Autodesk Inventor part; units mm, degrees
(part 4 of 5)
  line L745 (-387.1432, 38.3282) -> (-386.5943, 38.3282)
  spline S682 degree 2 poles (-383.8413, 38.4244) (-383.8923, 38.447) (-384.0677, 38.4838) (-384.1243, 38.4838) knots 0 0 0 1 2 2 2
  spline S683 degree 2 poles (-384.1243, 38.4838) (-384.5741, 38.4838) (-384.5741, 37.9661) knots 0 0 0 1 1 1
  line L746 (-384.5741, 37.9661) -> (-384.5741, 37.0211)
  line L747 (-384.5741, 37.0211) -> (-385.4795, 37.0211)
  line L748 (-385.4795, 37.0211) -> (-385.4795, 39.1996)
  line L749 (-385.4795, 39.1996) -> (-384.5741, 39.1996)
  line L750 (-384.5741, 39.1996) -> (-384.5741, 38.8177)
  line L751 (-384.5741, 38.8177) -> (-384.5657, 38.8177)
  spline S684 degree 2 poles (-384.5657, 38.8177) (-384.4836, 39.0242) (-384.1752, 39.2392) (-383.9715, 39.2392) knots 0 0 0 1 2 2 2
  spline S685 degree 2 poles (-383.9715, 39.2392) (-383.8979, 39.2392) (-383.8413, 39.2138) knots 0 0 0 1 1 1
  line L752 (-383.8413, 39.2138) -> (-383.8413, 38.4244)
  spline S686 degree 2 poles (-381.9429, 38.4244) (-381.9938, 38.447) (-382.1692, 38.4838) (-382.2258, 38.4838) knots 0 0 0 1 2 2 2
  spline S687 degree 2 poles (-382.2258, 38.4838) (-382.6757, 38.4838) (-382.6757, 37.9661) knots 0 0 0 1 1 1
  line L753 (-382.6757, 37.9661) -> (-382.6757, 37.0211)
  line L754 (-382.6757, 37.0211) -> (-383.5811, 37.0211)
  line L755 (-383.5811, 37.0211) -> (-383.5811, 39.1996)
  line L756 (-383.5811, 39.1996) -> (-382.6757, 39.1996)
  line L757 (-382.6757, 39.1996) -> (-382.6757, 38.8177)
  line L758 (-382.6757, 38.8177) -> (-382.6672, 38.8177)
  spline S688 degree 2 poles (-382.6672, 38.8177) (-382.5851, 39.0242) (-382.2767, 39.2392) (-382.073, 39.2392) knots 0 0 0 1 2 2 2
  spline S689 degree 2 poles (-382.073, 39.2392) (-381.9995, 39.2392) (-381.9429, 39.2138) knots 0 0 0 1 1 1
  line L759 (-381.9429, 39.2138) -> (-381.9429, 38.4244)
  spline S690 degree 2 poles (-379.2607, 38.15) (-379.2607, 37.5982) (-379.9256, 36.9673) (-380.5226, 36.9673) knots 0 0 0 1 2 2 2
  spline S691 degree 2 poles (-380.5226, 36.9673) (-381.1167, 36.9673) (-381.7788, 37.5813) (-381.7788, 38.1245) knots 0 0 0 1 2 2 2
  spline S692 degree 2 poles (-381.7788, 38.1245) (-381.7788, 38.4697) (-381.4676, 38.9818) (-380.8932, 39.2534) (-380.5197, 39.2534) knots 0 0 0 1 2 3 3 3
  spline S693 degree 2 poles (-380.5197, 39.2534) (-380.1321, 39.2534) (-379.5634, 38.9676) (-379.2607, 38.4612) (-379.2607, 38.15) knots 0 0 0 1 2 3 3 3
  spline S694 degree 2 poles (-380.1802, 38.1443) (-380.1802, 38.5885) (-380.5197, 38.5885) knots 0 0 0 1 1 1
  spline S695 degree 2 poles (-380.5197, 38.5885) (-380.8593, 38.5885) (-380.8593, 38.1245) knots 0 0 0 1 1 1
  spline S696 degree 2 poles (-380.8593, 38.1245) (-380.8593, 37.6322) (-380.5141, 37.6322) knots 0 0 0 1 1 1
  spline S697 degree 2 poles (-380.5141, 37.6322) (-380.1802, 37.6322) (-380.1802, 38.1443) knots 0 0 0 1 1 1
  line L760 (-380.6272, 39.5448) -> (-381.3855, 40.2267)
  line L761 (-381.3855, 40.2267) -> (-380.6244, 40.2267)
  line L762 (-380.6244, 40.2267) -> (-379.9878, 39.5448)
  line L763 (-379.9878, 39.5448) -> (-380.6272, 39.5448)
  line L764 (-376.7086, 39.3524) -> (-376.7086, 38.8035)
  line L765 (-376.7086, 38.8035) -> (-375.8033, 38.8035)
  line L766 (-375.8033, 38.8035) -> (-375.8033, 38.0849)
  line L767 (-375.8033, 38.0849) -> (-376.7086, 38.0849)
  line L768 (-376.7086, 38.0849) -> (-376.7086, 37.0211)
  line L769 (-376.7086, 37.0211) -> (-377.6282, 37.0211)
  line L770 (-377.6282, 37.0211) -> (-377.6282, 40.0711)
  line L771 (-377.6282, 40.0711) -> (-375.7156, 40.0711)
  line L772 (-375.7156, 40.0711) -> (-375.7156, 39.3524)
  line L773 (-375.7156, 39.3524) -> (-376.7086, 39.3524)
  spline S698 degree 2 poles (-373.7152, 38.4244) (-373.7662, 38.447) (-373.9416, 38.4838) (-373.9982, 38.4838) knots 0 0 0 1 2 2 2
  spline S699 degree 2 poles (-373.9982, 38.4838) (-374.448, 38.4838) (-374.448, 37.9661) knots 0 0 0 1 1 1
  line L774 (-374.448, 37.9661) -> (-374.448, 37.0211)
  line L775 (-374.448, 37.0211) -> (-375.3534, 37.0211)
  line L776 (-375.3534, 37.0211) -> (-375.3534, 39.1996)
  line L777 (-375.3534, 39.1996) -> (-374.448, 39.1996)
  line L778 (-374.448, 39.1996) -> (-374.448, 38.8177)
  line L779 (-374.448, 38.8177) -> (-374.4395, 38.8177)
  spline S700 degree 2 poles (-374.4395, 38.8177) (-374.3575, 39.0242) (-374.0491, 39.2392) (-373.8454, 39.2392) knots 0 0 0 1 2 2 2
  spline S701 degree 2 poles (-373.8454, 39.2392) (-373.7718, 39.2392) (-373.7152, 39.2138) knots 0 0 0 1 1 1
  line L780 (-373.7152, 39.2138) -> (-373.7152, 38.4244)
  line L781 (-372.2468, 37.0211) -> (-372.2468, 37.3521)
  line L782 (-372.2468, 37.3521) -> (-372.2553, 37.3521)
  spline S702 degree 2 poles (-372.2553, 37.3521) (-372.4732, 36.9673) (-372.9202, 36.9673) knots 0 0 0 1 1 1
  spline S703 degree 2 poles (-372.9202, 36.9673) (-373.2286, 36.9673) (-373.5766, 37.3323) (-373.5766, 37.6407) knots 0 0 0 1 2 2 2
  spline S704 degree 2 poles (-373.5766, 37.6407) (-373.5766, 38.2829) (-372.7872, 38.3848) knots 0 0 0 1 1 1
  line L783 (-372.7872, 38.3848) -> (-372.2468, 38.4555)
  spline S705 degree 2 poles (-372.2468, 38.4555) (-372.2468, 38.563) (-372.4392, 38.6988) (-372.6005, 38.6988) knots 0 0 0 1 2 2 2
  spline S706 degree 2 poles (-372.6005, 38.6988) (-372.9655, 38.6988) (-373.3729, 38.4895) knots 0 0 0 1 1 1
  line L784 (-373.3729, 38.4895) -> (-373.3729, 39.078)
  spline S707 degree 2 poles (-373.3729, 39.078) (-373.1975, 39.1544) (-372.6627, 39.2534) (-372.4732, 39.2534) knots 0 0 0 1 2 2 2
  spline S708 degree 2 poles (-372.4732, 39.2534) (-371.9186, 39.2534) (-371.4178, 38.7781) (-371.4178, 38.2235) knots 0 0 0 1 2 2 2
  line L785 (-371.4178, 38.2235) -> (-371.4178, 37.0211)
  line L786 (-371.4178, 37.0211) -> (-372.2468, 37.0211)
  spline S709 degree 2 poles (-372.7844, 37.7623) (-372.7844, 37.6746) (-372.6712, 37.5586) (-372.5665, 37.5586) knots 0 0 0 1 2 2 2
  spline S710 degree 2 poles (-372.5665, 37.5586) (-372.4251, 37.5586) (-372.2468, 37.7708) (-372.2468, 37.9378) knots 0 0 0 1 2 2 2
  line L787 (-372.2468, 37.9378) -> (-372.2468, 38.0198)
  line L788 (-372.2468, 38.0198) -> (-372.5552, 37.9774)
  spline S711 degree 2 poles (-372.5552, 37.9774) (-372.7844, 37.9378) (-372.7844, 37.7623) knots 0 0 0 1 1 1
  line L789 (-369.5986, 37.0211) -> (-369.5986, 38.2094)
  spline S712 degree 2 poles (-369.5986, 38.2094) (-369.5986, 38.4131) (-369.7202, 38.5885) (-369.8561, 38.5885) knots 0 0 0 1 2 2 2
  spline S713 degree 2 poles (-369.8561, 38.5885) (-369.9721, 38.5885) (-370.105, 38.4046) (-370.105, 38.2631) knots 0 0 0 1 2 2 2
  line L790 (-370.105, 38.2631) -> (-370.105, 37.0211)
  line L791 (-370.105, 37.0211) -> (-371.0104, 37.0211)
  line L792 (-371.0104, 37.0211) -> (-371.0104, 39.1996)
  line L793 (-371.0104, 39.1996) -> (-370.105, 39.1996)
  line L794 (-370.105, 39.1996) -> (-370.105, 38.8601)
  line L795 (-370.105, 38.8601) -> (-370.0965, 38.8601)
  spline S714 degree 2 poles (-370.0965, 38.8601) (-369.989, 39.0469) (-369.6212, 39.2534) (-369.4062, 39.2534) knots 0 0 0 1 2 2 2
  spline S715 degree 2 poles (-369.4062, 39.2534) (-368.6932, 39.2534) (-368.6932, 38.3508) knots 0 0 0 1 1 1
  line L796 (-368.6932, 38.3508) -> (-368.6932, 37.0211)
  line L797 (-368.6932, 37.0211) -> (-369.5986, 37.0211)
  spline S716 degree 2 poles (-366.4892, 37.0833) (-366.5769, 37.0324) (-366.9503, 36.9673) (-367.1937, 36.9673) knots 0 0 0 1 2 2 2
  spline S717 degree 2 poles (-367.1937, 36.9673) (-367.5388, 36.9673) (-368.0821, 37.2474) (-368.3791, 37.7482) (-368.3791, 38.0622) knots 0 0 0 1 2 3 3 3
  spline S718 degree 2 poles (-368.3791, 38.0622) (-368.3791, 38.4357) (-368.0623, 38.9705) (-367.4766, 39.2534) (-367.089, 39.2534) knots 0 0 0 1 2 3 3 3
  spline S719 degree 2 poles (-367.089, 39.2534) (-366.8768, 39.2534) (-366.5373, 39.1968) (-366.4892, 39.1629) knots 0 0 0 1 2 2 2
  line L798 (-366.4892, 39.1629) -> (-366.4892, 38.4555)
  spline S720 degree 2 poles (-366.4892, 38.4555) (-366.5571, 38.5093) (-366.8117, 38.5885) (-366.9192, 38.5885) knots 0 0 0 1 2 2 2
  spline S721 degree 2 poles (-366.9192, 38.5885) (-367.1852, 38.5885) (-367.4596, 38.3367) (-367.4596, 38.1075) knots 0 0 0 1 2 2 2
  spline S722 degree 2 poles (-367.4596, 38.1075) (-367.4596, 37.8812) (-367.1908, 37.6322) (-366.9532, 37.6322) knots 0 0 0 1 2 2 2
  spline S723 degree 2 poles (-366.9532, 37.6322) (-366.7014, 37.6322) (-366.4892, 37.751) knots 0 0 0 1 1 1
  line L799 (-366.4892, 37.751) -> (-366.4892, 37.0833)
  spline S724 degree 2 poles (-365.3461, 37.8529) (-365.3235, 37.7114) (-365.0462, 37.553) (-364.8199, 37.553) knots 0 0 0 1 2 2 2
  spline S725 degree 2 poles (-364.8199, 37.553) (-364.503, 37.553) (-364.2201, 37.6746) knots 0 0 0 1 1 1
  line L800 (-364.2201, 37.6746) -> (-364.2201, 37.1003)
  spline S726 degree 2 poles (-364.2201, 37.1003) (-364.5483, 36.9673) (-365.0208, 36.9673) knots 0 0 0 1 1 1
  spline S727 degree 2 poles (-365.0208, 36.9673) (-365.5894, 36.9673) (-366.2232, 37.5501) (-366.2232, 38.0622) knots 0 0 0 1 2 2 2
  spline S728 degree 2 poles (-366.2232, 38.0622) (-366.2232, 38.4131) (-365.9459, 38.9478) (-365.3999, 39.2534) (-365.0689, 39.2534) knots 0 0 0 1 2 3 3 3
  spline S729 degree 2 poles (-365.0689, 39.2534) (-364.7322, 39.2534) (-364.2512, 38.9903) (-364.0022, 38.5121) (-364.0022, 38.1924) knots 0 0 0 1 2 3 3 3
  line L801 (-364.0022, 38.1924) -> (-364.0022, 37.8529)
  line L802 (-364.0022, 37.8529) -> (-365.3461, 37.8529)
  spline S730 degree 2 poles (-364.8029, 38.3282) (-364.8029, 38.7045) (-365.0717, 38.7045) knots 0 0 0 1 1 1
  spline S731 degree 2 poles (-365.0717, 38.7045) (-365.1849, 38.7045) (-365.3376, 38.498) (-365.3518, 38.3282) knots 0 0 0 1 2 2 2
  line L803 (-365.3518, 38.3282) -> (-364.8029, 38.3282)
  spline S732 degree 2 poles (-361.917, 37.7454) (-361.917, 37.3747) (-362.4829, 36.9673) (-362.9865, 36.9673) knots 0 0 0 1 2 2 2
  spline S733 degree 2 poles (-362.9865, 36.9673) (-363.1336, 36.9673) (-363.5665, 37.0267) (-363.7023, 37.0692) knots 0 0 0 1 2 2 2
  line L804 (-363.7023, 37.0692) -> (-363.7023, 37.7058)
  spline S734 degree 2 poles (-363.7023, 37.7058) (-363.3005, 37.5275) (-363.0289, 37.5275) knots 0 0 0 1 1 1
  spline S735 degree 2 poles (-363.0289, 37.5275) (-362.763, 37.5275) (-362.763, 37.6661) knots 0 0 0 1 1 1
  spline S736 degree 2 poles (-362.763, 37.6661) (-362.763, 37.7227) (-362.8875, 37.7991) (-363.1477, 37.884) knots 0 0 0 1 2 2 2
  spline S737 degree 2 poles (-363.1477, 37.884) (-363.4392, 37.9774) (-363.7023, 38.2801) (-363.7023, 38.5206) knots 0 0 0 1 2 2 2
  spline S738 degree 2 poles (-363.7023, 38.5206) (-363.7023, 38.8601) (-363.1619, 39.2534) (-362.6753, 39.2534) knots 0 0 0 1 2 2 2
  spline S739 degree 2 poles (-362.6753, 39.2534) (-362.3895, 39.2534) (-362.0698, 39.1713) knots 0 0 0 1 1 1
  line L805 (-362.0698, 39.1713) -> (-362.0698, 38.5602)
  spline S740 degree 2 poles (-362.0698, 38.5602) (-362.2056, 38.6168) (-362.5253, 38.6932) (-362.6328, 38.6932) knots 0 0 0 1 2 2 2
  spline S741 degree 2 poles (-362.6328, 38.6932) (-362.7234, 38.6932) (-362.8309, 38.6338) (-362.8309, 38.58) knots 0 0 0 1 2 2 2
  spline S742 degree 2 poles (-362.8309, 38.58) (-362.8309, 38.5178) (-362.7149, 38.4414) (-362.5423, 38.3876) knots 0 0 0 1 2 2 2
  spline S743 degree 2 poles (-362.5423, 38.3876) (-362.2084, 38.2914) (-361.917, 37.9859) (-361.917, 37.7454) knots 0 0 0 1 2 2 2
  spline S744 degree 2 poles (-359.7894, 37.0833) (-359.8771, 37.0324) (-360.2505, 36.9673) (-360.4939, 36.9673) knots 0 0 0 1 2 2 2
  spline S745 degree 2 poles (-360.4939, 36.9673) (-360.839, 36.9673) (-361.3823, 37.2474) (-361.6793, 37.7482) (-361.6793, 38.0622) knots 0 0 0 1 2 3 3 3
  spline S746 degree 2 poles (-361.6793, 38.0622) (-361.6793, 38.4357) (-361.3625, 38.9705) (-360.7768, 39.2534) (-360.3892, 39.2534) knots 0 0 0 1 2 3 3 3
  spline S747 degree 2 poles (-360.3892, 39.2534) (-360.177, 39.2534) (-359.8375, 39.1968) (-359.7894, 39.1629) knots 0 0 0 1 2 2 2
  line L806 (-359.7894, 39.1629) -> (-359.7894, 38.4555)
  spline S748 degree 2 poles (-359.7894, 38.4555) (-359.8573, 38.5093) (-360.1119, 38.5885) (-360.2194, 38.5885) knots 0 0 0 1 2 2 2
  spline S749 degree 2 poles (-360.2194, 38.5885) (-360.4854, 38.5885) (-360.7598, 38.3367) (-360.7598, 38.1075) knots 0 0 0 1 2 2 2
  spline S750 degree 2 poles (-360.7598, 38.1075) (-360.7598, 37.8812) (-360.491, 37.6322) (-360.2534, 37.6322) knots 0 0 0 1 2 2 2
  spline S751 degree 2 poles (-360.2534, 37.6322) (-360.0016, 37.6322) (-359.7894, 37.751) knots 0 0 0 1 1 1
  line L807 (-359.7894, 37.751) -> (-359.7894, 37.0833)
  spline S752 degree 2 poles (-357.0053, 38.15) (-357.0053, 37.5982) (-357.6702, 36.9673) (-358.2672, 36.9673) knots 0 0 0 1 2 2 2
  spline S753 degree 2 poles (-358.2672, 36.9673) (-358.8613, 36.9673) (-359.5234, 37.5813) (-359.5234, 38.1245) knots 0 0 0 1 2 2 2
  spline S754 degree 2 poles (-359.5234, 38.1245) (-359.5234, 38.4697) (-359.2122, 38.9818) (-358.6378, 39.2534) (-358.2644, 39.2534) knots 0 0 0 1 2 3 3 3
  spline S755 degree 2 poles (-358.2644, 39.2534) (-357.8767, 39.2534) (-357.308, 38.9676) (-357.0053, 38.4612) (-357.0053, 38.15) knots 0 0 0 1 2 3 3 3
  spline S756 degree 2 poles (-357.9248, 38.1443) (-357.9248, 38.5885) (-358.2644, 38.5885) knots 0 0 0 1 1 1
  spline S757 degree 2 poles (-358.2644, 38.5885) (-358.6039, 38.5885) (-358.6039, 38.1245) knots 0 0 0 1 1 1
  spline S758 degree 2 poles (-358.6039, 38.1245) (-358.6039, 37.6322) (-358.2587, 37.6322) knots 0 0 0 1 1 1
  spline S759 degree 2 poles (-358.2587, 37.6322) (-357.9248, 37.6322) (-357.9248, 38.1443) knots 0 0 0 1 1 1
  spline S760 degree 2 poles (-268.9959, 67.4041) (-268.9959, 66.9542) (-269.6268, 66.4676) (-270.2097, 66.4676) knots 0 0 0 1 2 2 2
  line L808 (-270.2097, 66.4676) -> (-271.6017, 66.4676)
  line L809 (-271.6017, 66.4676) -> (-271.6017, 69.5176)
  line L810 (-271.6017, 69.5176) -> (-270.3059, 69.5176)
  spline S761 degree 2 poles (-270.3059, 69.5176) (-269.0921, 69.5176) (-269.0921, 68.7791) knots 0 0 0 1 1 1
  spline S762 degree 2 poles (-269.0921, 68.7791) (-269.0921, 68.6207) (-269.2449, 68.3547) (-269.5589, 68.1539) (-269.7457, 68.1171) knots 0 0 0 1 2 3 3 3
  line L811 (-269.7457, 68.1171) -> (-269.7457, 68.1086)
  spline S763 degree 2 poles (-269.7457, 68.1086) (-269.5278, 68.0831) (-269.1826, 67.8766) (-268.9959, 67.5682) (-268.9959, 67.4041) knots 0 0 0 1 2 3 3 3
  spline S764 degree 2 poles (-269.972, 67.4069) (-269.972, 67.5399) (-270.1644, 67.7097) (-270.32, 67.7097) knots 0 0 0 1 2 2 2
  line L812 (-270.32, 67.7097) -> (-270.6822, 67.7097)
  line L813 (-270.6822, 67.7097) -> (-270.6822, 67.0872)
  line L814 (-270.6822, 67.0872) -> (-270.3766, 67.0872)
  spline S765 degree 2 poles (-270.3766, 67.0872) (-270.1899, 67.0872) (-269.972, 67.2598) (-269.972, 67.4069) knots 0 0 0 1 2 2 2
  spline S766 degree 2 poles (-270.0682, 68.6207) (-270.0682, 68.9036) (-270.5124, 68.9036) knots 0 0 0 1 1 1
  line L815 (-270.5124, 68.9036) -> (-270.6822, 68.9036)
  line L816 (-270.6822, 68.9036) -> (-270.6822, 68.3264)
  line L817 (-270.6822, 68.3264) -> (-270.4162, 68.3264)
  spline S767 degree 2 poles (-270.4162, 68.3264) (-270.2634, 68.3264) (-270.0682, 68.4905) (-270.0682, 68.6207) knots 0 0 0 1 2 2 2
  spline S768 degree 2 poles (-266.2515, 67.5965) (-266.2515, 67.0448) (-266.9163, 66.4138) (-267.5133, 66.4138) knots 0 0 0 1 2 2 2
  spline S769 degree 2 poles (-267.5133, 66.4138) (-268.1075, 66.4138) (-268.7695, 67.0278) (-268.7695, 67.571) knots 0 0 0 1 2 2 2
  spline S770 degree 2 poles (-268.7695, 67.571) (-268.7695, 67.9162) (-268.4583, 68.4283) (-267.884, 68.6999) (-267.5105, 68.6999) knots 0 0 0 1 2 3 3 3
  spline S771 degree 2 poles (-267.5105, 68.6999) (-267.1229, 68.6999) (-266.5542, 68.4142) (-266.2515, 67.9077) (-266.2515, 67.5965) knots 0 0 0 1 2 3 3 3
  spline S772 degree 2 poles (-267.171, 67.5908) (-267.171, 68.035) (-267.5105, 68.035) knots 0 0 0 1 1 1
  spline S773 degree 2 poles (-267.5105, 68.035) (-267.85, 68.035) (-267.85, 67.571) knots 0 0 0 1 1 1
  spline S774 degree 2 poles (-267.85, 67.571) (-267.85, 67.0787) (-267.5048, 67.0787) knots 0 0 0 1 1 1
  spline S775 degree 2 poles (-267.5048, 67.0787) (-267.171, 67.0787) (-267.171, 67.5908) knots 0 0 0 1 1 1
  line L818 (-264.7038, 66.4676) -> (-264.7038, 66.7986)
  line L819 (-264.7038, 66.7986) -> (-264.7123, 66.7986)
  spline S776 degree 2 poles (-264.7123, 66.7986) (-264.9302, 66.4138) (-265.3772, 66.4138) knots 0 0 0 1 1 1
  spline S777 degree 2 poles (-265.3772, 66.4138) (-265.6856, 66.4138) (-266.0336, 66.7788) (-266.0336, 67.0872) knots 0 0 0 1 2 2 2
  spline S778 degree 2 poles (-266.0336, 67.0872) (-266.0336, 67.7295) (-265.2442, 67.8313) knots 0 0 0 1 1 1
  line L820 (-265.2442, 67.8313) -> (-264.7038, 67.902)
  spline S779 degree 2 poles (-264.7038, 67.902) (-264.7038, 68.0096) (-264.8962, 68.1454) (-265.0575, 68.1454) knots 0 0 0 1 2 2 2
  spline S780 degree 2 poles (-265.0575, 68.1454) (-265.4225, 68.1454) (-265.8299, 67.936) knots 0 0 0 1 1 1
  line L821 (-265.8299, 67.936) -> (-265.8299, 68.5245)
  spline S781 degree 2 poles (-265.8299, 68.5245) (-265.6545, 68.6009) (-265.1197, 68.6999) (-264.9302, 68.6999) knots 0 0 0 1 2 2 2
  spline S782 degree 2 poles (-264.9302, 68.6999) (-264.3756, 68.6999) (-263.8748, 68.2246) (-263.8748, 67.67) knots 0 0 0 1 2 2 2
  line L822 (-263.8748, 67.67) -> (-263.8748, 66.4676)
  line L823 (-263.8748, 66.4676) -> (-264.7038, 66.4676)
  spline S783 degree 2 poles (-265.2414, 67.2089) (-265.2414, 67.1212) (-265.1282, 67.0052) (-265.0235, 67.0052) knots 0 0 0 1 2 2 2
  spline S784 degree 2 poles (-265.0235, 67.0052) (-264.8821, 67.0052) (-264.7038, 67.2174) (-264.7038, 67.3843) knots 0 0 0 1 2 2 2
  line L824 (-264.7038, 67.3843) -> (-264.7038, 67.4663)
  line L825 (-264.7038, 67.4663) -> (-265.0122, 67.4239)
  spline S785 degree 2 poles (-265.0122, 67.4239) (-265.2414, 67.3843) (-265.2414, 67.2089) knots 0 0 0 1 1 1
  spline S786 degree 2 poles (-261.8292, 67.8709) (-261.8802, 67.8936) (-262.0556, 67.9303) (-262.1122, 67.9303) knots 0 0 0 1 2 2 2
  spline S787 degree 2 poles (-262.1122, 67.9303) (-262.562, 67.9303) (-262.562, 67.4126) knots 0 0 0 1 1 1
  line L826 (-262.562, 67.4126) -> (-262.562, 66.4676)
  line L827 (-262.562, 66.4676) -> (-263.4674, 66.4676)
  line L828 (-263.4674, 66.4676) -> (-263.4674, 68.6462)
  line L829 (-263.4674, 68.6462) -> (-262.562, 68.6462)
  line L830 (-262.562, 68.6462) -> (-262.562, 68.2642)
  line L831 (-262.562, 68.2642) -> (-262.5535, 68.2642)
  spline S788 degree 2 poles (-262.5535, 68.2642) (-262.4715, 68.4707) (-262.1631, 68.6858) (-261.9594, 68.6858) knots 0 0 0 1 2 2 2
  spline S789 degree 2 poles (-261.9594, 68.6858) (-261.8858, 68.6858) (-261.8292, 68.6603) knots 0 0 0 1 1 1
  line L832 (-261.8292, 68.6603) -> (-261.8292, 67.8709)
  line L833 (-260.1147, 66.4676) -> (-260.1147, 66.7222)
  line L834 (-260.1147, 66.7222) -> (-260.1232, 66.7222)
  spline S790 degree 2 poles (-260.1232, 66.7222) (-260.2307, 66.5779) (-260.5815, 66.4138) (-260.7513, 66.4138) knots 0 0 0 1 2 2 2
  spline S791 degree 2 poles (-260.7513, 66.4138) (-261.0285, 66.4138) (-261.4558, 66.6883) (-261.6651, 67.1834) (-261.6651, 67.5173) knots 0 0 0 1 2 3 3 3
  spline S792 degree 2 poles (-261.6651, 67.5173) (-261.6651, 67.8653) (-261.4133, 68.4028) (-260.9578, 68.6999) (-260.6749, 68.6999) knots 0 0 0 1 2 3 3 3
  spline S793 degree 2 poles (-260.6749, 68.6999) (-260.5419, 68.6999) (-260.3156, 68.6235) (-260.1458, 68.4934) (-260.1232, 68.4283) knots 0 0 0 1 2 3 3 3
  line L835 (-260.1232, 68.4283) -> (-260.1147, 68.4283)
  line L836 (-260.1147, 68.4283) -> (-260.1147, 69.693)
  line L837 (-260.1147, 69.693) -> (-259.2093, 69.693)
  line L838 (-259.2093, 69.693) -> (-259.2093, 66.4676)
  line L839 (-259.2093, 66.4676) -> (-260.1147, 66.4676)
  spline S794 degree 2 poles (-260.0949, 67.6219) (-260.0949, 67.8172) (-260.2675, 68.035) (-260.4146, 68.035) knots 0 0 0 1 2 2 2
  spline S795 degree 2 poles (-260.4146, 68.035) (-260.5617, 68.035) (-260.7456, 67.7662) (-260.7456, 67.5399) knots 0 0 0 1 2 2 2
  spline S796 degree 2 poles (-260.7456, 67.5399) (-260.7456, 67.0787) (-260.4259, 67.0787) knots 0 0 0 1 1 1
  spline S797 degree 2 poles (-260.4259, 67.0787) (-260.2759, 67.0787) (-260.0949, 67.3277) (-260.0949, 67.5654) knots 0 0 0 1 2 2 2
  line L840 (-260.0949, 67.5654) -> (-260.0949, 67.6219)
  line L841 (-255.4774, 66.4619) -> (-255.6557, 66.6713)
  spline S798 degree 2 poles (-255.6557, 66.6713) (-255.7971, 66.5609) (-256.3121, 66.4138) (-256.5469, 66.4138) knots 0 0 0 1 2 2 2
  spline S799 degree 2 poles (-256.5469, 66.4138) (-257.0675, 66.4138) (-257.6475, 66.8665) (-257.6475, 67.2739) knots 0 0 0 1 2 2 2
  spline S800 degree 2 poles (-257.6475, 67.2739) (-257.6475, 67.5144) (-257.2995, 67.953) (-256.9402, 68.1312) knots 0 0 0 1 2 2 2
  spline S801 degree 2 poles (-256.9402, 68.1312) (-257.2458, 68.4679) (-257.2458, 68.8018) knots 0 0 0 1 1 1
  spline S802 degree 2 poles (-257.2458, 68.8018) (-257.2458, 69.1441) (-256.711, 69.5685) (-256.2838, 69.5685) knots 0 0 0 1 2 2 2
  spline S803 degree 2 poles (-256.2838, 69.5685) (-255.8764, 69.5685) (-255.3812, 69.1866) (-255.3812, 68.8697) knots 0 0 0 1 2 2 2
  spline S804 degree 2 poles (-255.3812, 68.8697) (-255.3812, 68.6179) (-255.6755, 68.2529) (-255.9924, 68.1058) knots 0 0 0 1 2 2 2
  line L842 (-255.9924, 68.1058) -> (-255.5595, 67.6135)
  spline S805 degree 2 poles (-255.5595, 67.6135) (-255.4633, 67.8058) (-255.4633, 68.1312) knots 0 0 0 1 1 1
  line L843 (-255.4633, 68.1312) -> (-254.7701, 68.1312)
  spline S806 degree 2 poles (-254.7701, 68.1312) (-254.7701, 67.8228) (-254.9455, 67.3305) (-255.1407, 67.1268) knots 0 0 0 1 2 2 2
  line L844 (-255.1407, 67.1268) -> (-254.5296, 66.4619)
  line L845 (-254.5296, 66.4619) -> (-255.4774, 66.4619)
  spline S807 degree 2 poles (-256.6205, 67.7606) (-256.711, 67.7181) (-256.8327, 67.5088) (-256.8327, 67.3786) knots 0 0 0 1 2 2 2
  spline S808 degree 2 poles (-256.8327, 67.3786) (-256.8327, 67.1975) (-256.5922, 66.9769) (-256.4168, 66.9769) knots 0 0 0 1 2 2 2
  spline S809 degree 2 poles (-256.4168, 66.9769) (-256.3093, 66.9769) (-256.1055, 67.0476) (-256.0376, 67.1042) knots 0 0 0 1 2 2 2
  line L846 (-256.0376, 67.1042) -> (-256.6205, 67.7606)
  spline S810 degree 2 poles (-256.0801, 68.8244) (-256.0801, 68.9149) (-256.2131, 69.0451) (-256.3036, 69.0451) knots 0 0 0 1 2 2 2
  spline S811 degree 2 poles (-256.3036, 69.0451) (-256.4111, 69.0451) (-256.5384, 68.9291) (-256.5384, 68.8272) knots 0 0 0 1 2 2 2
  spline S812 degree 2 poles (-256.5384, 68.8272) (-256.5384, 68.7622) (-256.4592, 68.6235) (-256.3177, 68.4622) knots 0 0 0 1 2 2 2
  spline S813 degree 2 poles (-256.3177, 68.4622) (-256.1848, 68.5443) (-256.0801, 68.7141) (-256.0801, 68.8244) knots 0 0 0 1 2 2 2
  spline S814 degree 2 poles (-250.7779, 66.5496) (-251.1571, 66.4138) (-251.6522, 66.4138) knots 0 0 0 1 1 1
  spline S815 degree 2 poles (-251.6522, 66.4138) (-252.1388, 66.4138) (-252.8433, 66.7873) (-253.2168, 67.472) (-253.2168, 67.9218) knots 0 0 0 1 2 3 3 3
  spline S816 degree 2 poles (-253.2168, 67.9218) (-253.2168, 68.4057) (-252.8009, 69.1583) (-252.0398, 69.5685) (-251.5447, 69.5685) knots 0 0 0 1 2 3 3 3
  spline S817 degree 2 poles (-251.5447, 69.5685) (-251.1486, 69.5685) (-250.7779, 69.4723) knots 0 0 0 1 1 1
  line L847 (-250.7779, 69.4723) -> (-250.7779, 68.6235)
  spline S818 degree 2 poles (-250.7779, 68.6235) (-250.9053, 68.6999) (-251.2589, 68.7848) (-251.4372, 68.7848) knots 0 0 0 1 2 2 2
  spline S819 degree 2 poles (-251.4372, 68.7848) (-251.8135, 68.7848) (-252.2435, 68.3547) (-252.2435, 67.9869) knots 0 0 0 1 2 2 2
  spline S820 degree 2 poles (-252.2435, 67.9869) (-252.2435, 67.6219) (-251.8135, 67.1975) (-251.4513, 67.1975) knots 0 0 0 1 2 2 2
  spline S821 degree 2 poles (-251.4513, 67.1975) (-251.1175, 67.1975) (-250.7779, 67.3701) knots 0 0 0 1 1 1
  line L848 (-250.7779, 67.3701) -> (-250.7779, 66.5496)
  line L849 (-249.1766, 66.4676) -> (-249.1766, 66.7986)
  line L850 (-249.1766, 66.7986) -> (-249.185, 66.7986)
  spline S822 degree 2 poles (-249.185, 66.7986) (-249.4029, 66.4138) (-249.8499, 66.4138) knots 0 0 0 1 1 1
  spline S823 degree 2 poles (-249.8499, 66.4138) (-250.1583, 66.4138) (-250.5063, 66.7788) (-250.5063, 67.0872) knots 0 0 0 1 2 2 2
  spline S824 degree 2 poles (-250.5063, 67.0872) (-250.5063, 67.7295) (-249.717, 67.8313) knots 0 0 0 1 1 1
  line L851 (-249.717, 67.8313) -> (-249.1766, 67.902)
  spline S825 degree 2 poles (-249.1766, 67.902) (-249.1766, 68.0096) (-249.3689, 68.1454) (-249.5302, 68.1454) knots 0 0 0 1 2 2 2
  spline S826 degree 2 poles (-249.5302, 68.1454) (-249.8952, 68.1454) (-250.3026, 67.936) knots 0 0 0 1 1 1
  line L852 (-250.3026, 67.936) -> (-250.3026, 68.5245)
  spline S827 degree 2 poles (-250.3026, 68.5245) (-250.1272, 68.6009) (-249.5925, 68.6999) (-249.4029, 68.6999) knots 0 0 0 1 2 2 2
  spline S828 degree 2 poles (-249.4029, 68.6999) (-248.8484, 68.6999) (-248.3476, 68.2246) (-248.3476, 67.67) knots 0 0 0 1 2 2 2
  line L853 (-248.3476, 67.67) -> (-248.3476, 66.4676)
  line L854 (-248.3476, 66.4676) -> (-249.1766, 66.4676)
  spline S829 degree 2 poles (-249.7141, 67.2089) (-249.7141, 67.1212) (-249.6009, 67.0052) (-249.4963, 67.0052) knots 0 0 0 1 2 2 2
  spline S830 degree 2 poles (-249.4963, 67.0052) (-249.3548, 67.0052) (-249.1766, 67.2174) (-249.1766, 67.3843) knots 0 0 0 1 2 2 2
  line L855 (-249.1766, 67.3843) -> (-249.1766, 67.4663)
  line L856 (-249.1766, 67.4663) -> (-249.4849, 67.4239)
  spline S831 degree 2 poles (-249.4849, 67.4239) (-249.7141, 67.3843) (-249.7141, 67.2089) knots 0 0 0 1 1 1
  spline S832 degree 2 poles (-246.169, 67.1919) (-246.169, 66.8212) (-246.7349, 66.4138) (-247.2385, 66.4138) knots 0 0 0 1 2 2 2
  spline S833 degree 2 poles (-247.2385, 66.4138) (-247.3856, 66.4138) (-247.8185, 66.4732) (-247.9543, 66.5157) knots 0 0 0 1 2 2 2
  line L857 (-247.9543, 66.5157) -> (-247.9543, 67.1523)
  spline S834 degree 2 poles (-247.9543, 67.1523) (-247.5525, 66.974) (-247.2809, 66.974) knots 0 0 0 1 1 1
  spline S835 degree 2 poles (-247.2809, 66.974) (-247.015, 66.974) (-247.015, 67.1127) knots 0 0 0 1 1 1
  spline S836 degree 2 poles (-247.015, 67.1127) (-247.015, 67.1693) (-247.1394, 67.2456) (-247.3997, 67.3305) knots 0 0 0 1 2 2 2
  spline S837 degree 2 poles (-247.3997, 67.3305) (-247.6912, 67.4239) (-247.9543, 67.7266) (-247.9543, 67.9671) knots 0 0 0 1 2 2 2
  spline S838 degree 2 poles (-247.9543, 67.9671) (-247.9543, 68.3066) (-247.4139, 68.6999) (-246.9272, 68.6999) knots 0 0 0 1 2 2 2
  spline S839 degree 2 poles (-246.9272, 68.6999) (-246.6415, 68.6999) (-246.3218, 68.6179) knots 0 0 0 1 1 1
  line L858 (-246.3218, 68.6179) -> (-246.3218, 68.0067)
  spline S840 degree 2 poles (-246.3218, 68.0067) (-246.4576, 68.0633) (-246.7773, 68.1397) (-246.8848, 68.1397) knots 0 0 0 1 2 2 2
  spline S841 degree 2 poles (-246.8848, 68.1397) (-246.9753, 68.1397) (-247.0829, 68.0803) (-247.0829, 68.0265) knots 0 0 0 1 2 2 2
  spline S842 degree 2 poles (-247.0829, 68.0265) (-247.0829, 67.9643) (-246.9669, 67.8879) (-246.7943, 67.8341) knots 0 0 0 1 2 2 2
  spline S843 degree 2 poles (-246.7943, 67.8341) (-246.4604, 67.7379) (-246.169, 67.4324) (-246.169, 67.1919) knots 0 0 0 1 2 2 2
  spline S844 degree 2 poles (-245.0542, 67.2994) (-245.0316, 67.1579) (-244.7543, 66.9995) (-244.528, 66.9995) knots 0 0 0 1 2 2 2
  spline S845 degree 2 poles (-244.528, 66.9995) (-244.2111, 66.9995) (-243.9282, 67.1212) knots 0 0 0 1 1 1
  line L859 (-243.9282, 67.1212) -> (-243.9282, 66.5468)
  spline S846 degree 2 poles (-243.9282, 66.5468) (-244.2564, 66.4138) (-244.7289, 66.4138) knots 0 0 0 1 1 1
  spline S847 degree 2 poles (-244.7289, 66.4138) (-245.2976, 66.4138) (-245.9313, 66.9967) (-245.9313, 67.5088) knots 0 0 0 1 2 2 2
  spline S848 degree 2 poles (-245.9313, 67.5088) (-245.9313, 67.8596) (-245.6541, 68.3943) (-245.108, 68.6999) (-244.777, 68.6999) knots 0 0 0 1 2 3 3 3
  spline S849 degree 2 poles (-244.777, 68.6999) (-244.4403, 68.6999) (-243.9593, 68.4368) (-243.7103, 67.9586) (-243.7103, 67.6389) knots 0 0 0 1 2 3 3 3
  line L860 (-243.7103, 67.6389) -> (-243.7103, 67.2994)
  line L861 (-243.7103, 67.2994) -> (-245.0542, 67.2994)
  spline S850 degree 2 poles (-244.511, 67.7747) (-244.511, 68.151) (-244.7798, 68.151) knots 0 0 0 1 1 1
  spline S851 degree 2 poles (-244.7798, 68.151) (-244.893, 68.151) (-245.0458, 67.9445) (-245.0599, 67.7747) knots 0 0 0 1 2 2 2
  line L862 (-245.0599, 67.7747) -> (-244.511, 67.7747)
  spline S852 degree 2 poles (-239.2259, 68.0322) (-239.2259, 67.5682) (-239.6163, 66.8552) (-240.3378, 66.4676) (-240.8103, 66.4676) knots 0 0 0 1 2 3 3 3
  line L863 (-240.8103, 66.4676) -> (-242.1033, 66.4676)
  line L864 (-242.1033, 66.4676) -> (-242.1033, 69.5176)
  line L865 (-242.1033, 69.5176) -> (-240.8386, 69.5176)
  spline S853 degree 2 poles (-240.8386, 69.5176) (-239.2259, 69.5176) (-239.2259, 68.0322) knots 0 0 0 1 1 1
  spline S854 degree 2 poles (-240.202, 68.0237) (-240.202, 68.2444) (-240.383, 68.6037) (-240.7197, 68.7989) (-240.9461, 68.7989) knots 0 0 0 1 2 3 3 3
  line L866 (-240.9461, 68.7989) -> (-241.1837, 68.7989)
  line L867 (-241.1837, 68.7989) -> (-241.1837, 67.1862)
  line L868 (-241.1837, 67.1862) -> (-240.9263, 67.1862)
  spline S855 degree 2 poles (-240.9263, 67.1862) (-240.5952, 67.1862) (-240.202, 67.6389) (-240.202, 68.0237) knots 0 0 0 1 2 2 2
  spline S856 degree 2 poles (-238.097, 67.2994) (-238.0743, 67.1579) (-237.7971, 66.9995) (-237.5707, 66.9995) knots 0 0 0 1 2 2 2
  spline S857 degree 2 poles (-237.5707, 66.9995) (-237.2538, 66.9995) (-236.9709, 67.1212) knots 0 0 0 1 1 1
  line L869 (-236.9709, 67.1212) -> (-236.9709, 66.5468)
  spline S858 degree 2 poles (-236.9709, 66.5468) (-237.2991, 66.4138) (-237.7716, 66.4138) knots 0 0 0 1 1 1
  spline S859 degree 2 poles (-237.7716, 66.4138) (-238.3403, 66.4138) (-238.974, 66.9967) (-238.974, 67.5088) knots 0 0 0 1 2 2 2
  spline S860 degree 2 poles (-238.974, 67.5088) (-238.974, 67.8596) (-238.6968, 68.3943) (-238.1507, 68.6999) (-237.8197, 68.6999) knots 0 0 0 1 2 3 3 3
  spline S861 degree 2 poles (-237.8197, 68.6999) (-237.483, 68.6999) (-237.002, 68.4368) (-236.753, 67.9586) (-236.753, 67.6389) knots 0 0 0 1 2 3 3 3
  line L870 (-236.753, 67.6389) -> (-236.753, 67.2994)
  line L871 (-236.753, 67.2994) -> (-238.097, 67.2994)
  spline S862 degree 2 poles (-237.5537, 67.7747) (-237.5537, 68.151) (-237.8225, 68.151) knots 0 0 0 1 1 1
  spline S863 degree 2 poles (-237.8225, 68.151) (-237.9357, 68.151) (-238.0885, 67.9445) (-238.1026, 67.7747) knots 0 0 0 1 2 2 2
  line L872 (-238.1026, 67.7747) -> (-237.5537, 67.7747)
  line L873 (-234.8546, 66.4676) -> (-235.9297, 66.4676)
  line L874 (-235.9297, 66.4676) -> (-236.6568, 68.6462)
  line L875 (-236.6568, 68.6462) -> (-235.7118, 68.6462)
  line L876 (-235.7118, 68.6462) -> (-235.4459, 67.4578)
  spline S864 degree 2 poles (-235.4459, 67.4578) (-235.3836, 67.1693) (-235.3752, 67.025) knots 0 0 0 1 1 1
  line L877 (-235.3752, 67.025) -> (-235.3638, 67.025)
  spline S865 degree 2 poles (-235.3638, 67.025) (-235.3582, 67.0674) (-235.344, 67.1579) (-235.0356, 68.6462) knots 0 0 0 1 2 2 2
  line L878 (-235.0356, 68.6462) -> (-234.0963, 68.6462)
  line L879 (-234.0963, 68.6462) -> (-234.8546, 66.4676)
  spline S866 degree 2 poles (-233.0976, 67.2994) (-233.0749, 67.1579) (-232.7977, 66.9995) (-232.5713, 66.9995) knots 0 0 0 1 2 2 2
  spline S867 degree 2 poles (-232.5713, 66.9995) (-232.2544, 66.9995) (-231.9715, 67.1212) knots 0 0 0 1 1 1
  line L880 (-231.9715, 67.1212) -> (-231.9715, 66.5468)
  spline S868 degree 2 poles (-231.9715, 66.5468) (-232.2997, 66.4138) (-232.7722, 66.4138) knots 0 0 0 1 1 1
  spline S869 degree 2 poles (-232.7722, 66.4138) (-233.3409, 66.4138) (-233.9746, 66.9967) (-233.9746, 67.5088) knots 0 0 0 1 2 2 2
  spline S870 degree 2 poles (-233.9746, 67.5088) (-233.9746, 67.8596) (-233.6974, 68.3943) (-233.1513, 68.6999) (-232.8203, 68.6999) knots 0 0 0 1 2 3 3 3
  spline S871 degree 2 poles (-232.8203, 68.6999) (-232.4836, 68.6999) (-232.0026, 68.4368) (-231.7536, 67.9586) (-231.7536, 67.6389) knots 0 0 0 1 2 3 3 3
  line L881 (-231.7536, 67.6389) -> (-231.7536, 67.2994)
  line L882 (-231.7536, 67.2994) -> (-233.0976, 67.2994)
  spline S872 degree 2 poles (-232.5543, 67.7747) (-232.5543, 68.151) (-232.8231, 68.151) knots 0 0 0 1 1 1
  spline S873 degree 2 poles (-232.8231, 68.151) (-232.9363, 68.151) (-233.0891, 67.9445) (-233.1032, 67.7747) knots 0 0 0 1 2 2 2
  line L883 (-233.1032, 67.7747) -> (-232.5543, 67.7747)
  line L884 (-231.4396, 66.4676) -> (-231.4396, 69.693)
  line L885 (-231.4396, 69.693) -> (-230.5342, 69.693)
  line L886 (-230.5342, 69.693) -> (-230.5342, 66.4676)
  line L887 (-230.5342, 66.4676) -> (-231.4396, 66.4676)
  spline S874 degree 2 poles (-227.6766, 67.5965) (-227.6766, 67.0448) (-228.3415, 66.4138) (-228.9385, 66.4138) knots 0 0 0 1 2 2 2
  spline S875 degree 2 poles (-228.9385, 66.4138) (-229.5326, 66.4138) (-230.1947, 67.0278) (-230.1947, 67.571) knots 0 0 0 1 2 2 2
  spline S876 degree 2 poles (-230.1947, 67.571) (-230.1947, 67.9162) (-229.8835, 68.4283) (-229.3091, 68.6999) (-228.9356, 68.6999) knots 0 0 0 1 2 3 3 3
  spline S877 degree 2 poles (-228.9356, 68.6999) (-228.548, 68.6999) (-227.9793, 68.4142) (-227.6766, 67.9077) (-227.6766, 67.5965) knots 0 0 0 1 2 3 3 3
  spline S878 degree 2 poles (-228.5961, 67.5908) (-228.5961, 68.035) (-228.9356, 68.035) knots 0 0 0 1 1 1
  spline S879 degree 2 poles (-228.9356, 68.035) (-229.2752, 68.035) (-229.2752, 67.571) knots 0 0 0 1 1 1
  spline S880 degree 2 poles (-229.2752, 67.571) (-229.2752, 67.0787) (-228.93, 67.0787) knots 0 0 0 1 1 1
  spline S881 degree 2 poles (-228.93, 67.0787) (-228.5961, 67.0787) (-228.5961, 67.5908) knots 0 0 0 1 1 1
  spline S882 degree 2 poles (-224.8812, 67.6219) (-224.8812, 67.2654) (-225.1246, 66.7166) (-225.5659, 66.4138) (-225.8432, 66.4138) knots 0 0 0 1 2 3 3 3
  spline S883 degree 2 poles (-225.8432, 66.4138) (-226.2252, 66.4138) (-226.4232, 66.6939) knots 0 0 0 1 1 1
  line L888 (-226.4232, 66.6939) -> (-226.4317, 66.6939)
  line L889 (-226.4317, 66.6939) -> (-226.4317, 65.466)
  line L890 (-226.4317, 65.466) -> (-227.3371, 65.466)
  line L891 (-227.3371, 65.466) -> (-227.3371, 68.6462)
  line L892 (-227.3371, 68.6462) -> (-226.4317, 68.6462)
  line L893 (-226.4317, 68.6462) -> (-226.4317, 68.3491)
  line L894 (-226.4317, 68.3491) -> (-226.4232, 68.3491)
  spline S884 degree 2 poles (-226.4232, 68.3491) (-226.3157, 68.5132) (-225.9705, 68.6999) (-225.7498, 68.6999) knots 0 0 0 1 2 2 2
  spline S885 degree 2 poles (-225.7498, 68.6999) (-225.3311, 68.6999) (-224.8812, 68.1369) (-224.8812, 67.6219) knots 0 0 0 1 2 2 2
  spline S886 degree 2 poles (-225.8008, 67.5965) (-225.8008, 67.8002) (-225.9592, 68.035) (-226.1261, 68.035) knots 0 0 0 1 2 2 2
  spline S887 degree 2 poles (-226.1261, 68.035) (-226.2704, 68.035) (-226.4487, 67.7889) (-226.4487, 67.5738) knots 0 0 0 1 2 2 2
  line L895 (-226.4487, 67.5738) -> (-226.4487, 67.5314)
  spline S888 degree 2 poles (-226.4487, 67.5314) (-226.4487, 67.3249) (-226.2959, 67.0787) (-226.1431, 67.0787) knots 0 0 0 1 2 2 2
  spline S889 degree 2 poles (-226.1431, 67.0787) (-225.979, 67.0787) (-225.8008, 67.3475) (-225.8008, 67.5965) knots 0 0 0 1 2 2 2
  spline S890 degree 2 poles (-223.758, 67.2994) (-223.7354, 67.1579) (-223.4581, 66.9995) (-223.2317, 66.9995) knots 0 0 0 1 2 2 2
  spline S891 degree 2 poles (-223.2317, 66.9995) (-222.9149, 66.9995) (-222.6319, 67.1212) knots 0 0 0 1 1 1
  line L896 (-222.6319, 67.1212) -> (-222.6319, 66.5468)
  spline S892 degree 2 poles (-222.6319, 66.5468) (-222.9601, 66.4138) (-223.4326, 66.4138) knots 0 0 0 1 1 1
  spline S893 degree 2 poles (-223.4326, 66.4138) (-224.0013, 66.4138) (-224.6351, 66.9967) (-224.6351, 67.5088) knots 0 0 0 1 2 2 2
  spline S894 degree 2 poles (-224.6351, 67.5088) (-224.6351, 67.8596) (-224.3578, 68.3943) (-223.8118, 68.6999) (-223.4807, 68.6999) knots 0 0 0 1 2 3 3 3
  spline S895 degree 2 poles (-223.4807, 68.6999) (-223.144, 68.6999) (-222.6631, 68.4368) (-222.4141, 67.9586) (-222.4141, 67.6389) knots 0 0 0 1 2 3 3 3
  line L897 (-222.4141, 67.6389) -> (-222.4141, 67.2994)
  line L898 (-222.4141, 67.2994) -> (-223.758, 67.2994)
  spline S896 degree 2 poles (-223.2148, 67.7747) (-223.2148, 68.151) (-223.4836, 68.151) knots 0 0 0 1 1 1
  spline S897 degree 2 poles (-223.4836, 68.151) (-223.5967, 68.151) (-223.7495, 67.9445) (-223.7637, 67.7747) knots 0 0 0 1 2 2 2
  line L899 (-223.7637, 67.7747) -> (-223.2148, 67.7747)
  line L900 (-220.6458, 66.4676) -> (-220.6458, 66.7222)
  line L901 (-220.6458, 66.7222) -> (-220.6542, 66.7222)
  spline S898 degree 2 poles (-220.6542, 66.7222) (-220.7618, 66.5779) (-221.1126, 66.4138) (-221.2823, 66.4138) knots 0 0 0 1 2 2 2
  spline S899 degree 2 poles (-221.2823, 66.4138) (-221.5596, 66.4138) (-221.9868, 66.6883) (-222.1962, 67.1834) (-222.1962, 67.5173) knots 0 0 0 1 2 3 3 3
  spline S900 degree 2 poles (-222.1962, 67.5173) (-222.1962, 67.8653) (-221.9444, 68.4028) (-221.4889, 68.6999) (-221.206, 68.6999) knots 0 0 0 1 2 3 3 3
  spline S901 degree 2 poles (-221.206, 68.6999) (-221.073, 68.6999) (-220.8466, 68.6235) (-220.6769, 68.4934) (-220.6542, 68.4283) knots 0 0 0 1 2 3 3 3
  line L902 (-220.6542, 68.4283) -> (-220.6458, 68.4283)
  line L903 (-220.6458, 68.4283) -> (-220.6458, 69.693)
  line L904 (-220.6458, 69.693) -> (-219.7404, 69.693)
  line L905 (-219.7404, 69.693) -> (-219.7404, 66.4676)
  line L906 (-219.7404, 66.4676) -> (-220.6458, 66.4676)
  spline S902 degree 2 poles (-220.6259, 67.6219) (-220.6259, 67.8172) (-220.7985, 68.035) (-220.9457, 68.035) knots 0 0 0 1 2 2 2
  spline S903 degree 2 poles (-220.9457, 68.035) (-221.0928, 68.035) (-221.2767, 67.7662) (-221.2767, 67.5399) knots 0 0 0 1 2 2 2
  spline S904 degree 2 poles (-221.2767, 67.5399) (-221.2767, 67.0787) (-220.957, 67.0787) knots 0 0 0 1 1 1
  spline S905 degree 2 poles (-220.957, 67.0787) (-220.807, 67.0787) (-220.6259, 67.3277) (-220.6259, 67.5654) knots 0 0 0 1 2 2 2
  line L907 (-220.6259, 67.5654) -> (-220.6259, 67.6219)
  spline S906 degree 2 poles (-215.635, 67.6219) (-215.635, 67.2654) (-215.8699, 66.7137) (-216.3056, 66.4138) (-216.58, 66.4138) knots 0 0 0 1 2 3 3 3
  spline S907 degree 2 poles (-216.58, 66.4138) (-216.7894, 66.4138) (-217.0893, 66.5694) (-217.177, 66.6939) knots 0 0 0 1 2 2 2
  line L908 (-217.177, 66.6939) -> (-217.1855, 66.6939)
  line L909 (-217.1855, 66.6939) -> (-217.1855, 66.4676)
  line L910 (-217.1855, 66.4676) -> (-218.0909, 66.4676)
  line L911 (-218.0909, 66.4676) -> (-218.0909, 69.693)
  line L912 (-218.0909, 69.693) -> (-217.1855, 69.693)
  line L913 (-217.1855, 69.693) -> (-217.1855, 68.3519)
  line L914 (-217.1855, 68.3519) -> (-217.177, 68.3519)
  spline S908 degree 2 poles (-217.177, 68.3519) (-217.0695, 68.5132) (-216.7073, 68.6999) (-216.4867, 68.6999) knots 0 0 0 1 2 2 2
  spline S909 degree 2 poles (-216.4867, 68.6999) (-216.0764, 68.6999) (-215.635, 68.151) (-215.635, 67.6219) knots 0 0 0 1 2 2 2
  spline S910 degree 2 poles (-216.5546, 67.5965) (-216.5546, 67.8143) (-216.7215, 68.035) (-216.8799, 68.035) knots 0 0 0 1 2 2 2
  spline S911 degree 2 poles (-216.8799, 68.035) (-217.0186, 68.035) (-217.2025, 67.803) (-217.2025, 67.6191) knots 0 0 0 1 2 2 2
  line L915 (-217.2025, 67.6191) -> (-217.2025, 67.4861)
  spline S912 degree 2 poles (-217.2025, 67.4861) (-217.2025, 67.2994) (-217.0355, 67.0787) (-216.8969, 67.0787) knots 0 0 0 1 2 2 2
  spline S913 degree 2 poles (-216.8969, 67.0787) (-216.7328, 67.0787) (-216.5546, 67.3475) (-216.5546, 67.5965) knots 0 0 0 1 2 2 2
  spline S914 degree 2 poles (-214.8711, 65.4434) (-214.9984, 65.4434) (-215.2899, 65.4886) (-215.4059, 65.5311) knots 0 0 0 1 2 2 2
  line L916 (-215.4059, 65.5311) -> (-215.4059, 66.2129)
  spline S915 degree 2 poles (-215.4059, 66.2129) (-215.3521, 66.1733) (-215.1427, 66.1054) (-215.0494, 66.1054) knots 0 0 0 1 2 2 2
  spline S916 degree 2 poles (-215.0494, 66.1054) (-214.7947, 66.1054) (-214.7127, 66.3063) knots 0 0 0 1 1 1
  line L917 (-214.7127, 66.3063) -> (-214.6419, 66.4761)
  line L918 (-214.6419, 66.4761) -> (-215.553, 68.6462)
  line L919 (-215.553, 68.6462) -> (-214.5514, 68.6462)
  line L920 (-214.5514, 68.6462) -> (-214.2883, 67.5965)
  spline S917 degree 2 poles (-214.2883, 67.5965) (-214.2119, 67.3022) (-214.2034, 67.2004) knots 0 0 0 1 1 1
  line L921 (-214.2034, 67.2004) -> (-214.1949, 67.2004)
  spline S918 degree 2 poles (-214.1949, 67.2004) (-214.1893, 67.2485) (-214.1666, 67.3616) (-213.8469, 68.6462) knots 0 0 0 1 2 2 2
  line L922 (-213.8469, 68.6462) -> (-212.967, 68.6462)
  line L923 (-212.967, 68.6462) -> (-213.7677, 66.4053)
  spline S919 degree 2 poles (-213.7677, 66.4053) (-213.9488, 65.8904) (-214.4835, 65.4434) (-214.8711, 65.4434) knots 0 0 0 1 2 2 2
  spline S920 degree 2 poles (-211.807, 66.8467) (-211.807, 66.6515) (-212.0786, 66.4138) (-212.3191, 66.4138) knots 0 0 0 1 2 2 2
  spline S921 degree 2 poles (-212.3191, 66.4138) (-212.5398, 66.4138) (-212.817, 66.6628) (-212.817, 66.8467) knots 0 0 0 1 2 2 2
  spline S922 degree 2 poles (-212.817, 66.8467) (-212.817, 67.0334) (-212.5426, 67.2654) (-212.3106, 67.2654) knots 0 0 0 1 2 2 2
  spline S923 degree 2 poles (-212.3106, 67.2654) (-212.0843, 67.2654) (-211.807, 67.0334) (-211.807, 66.8467) knots 0 0 0 1 2 2 2
  spline S924 degree 2 poles (-211.807, 68.2274) (-211.807, 68.0322) (-212.0814, 67.7974) (-212.3191, 67.7974) knots 0 0 0 1 2 2 2
  spline S925 degree 2 poles (-212.3191, 67.7974) (-212.5369, 67.7974) (-212.817, 68.0435) (-212.817, 68.2274) knots 0 0 0 1 2 2 2
  spline S926 degree 2 poles (-212.817, 68.2274) (-212.817, 68.4142) (-212.5426, 68.6462) (-212.3106, 68.6462) knots 0 0 0 1 2 2 2
  spline S927 degree 2 poles (-212.3106, 68.6462) (-212.0843, 68.6462) (-211.807, 68.4142) (-211.807, 68.2274) knots 0 0 0 1 2 2 2
  spline S928 degree 2 poles (-270.3285, 61.5693) (-270.3285, 61.4052) (-270.4983, 61.1138) (-270.7897, 60.9468) (-270.9509, 60.9468) knots 0 0 0 1 2 3 3 3
  spline S929 degree 2 poles (-270.9509, 60.9468) (-271.2028, 60.9468) (-271.5649, 61.309) (-271.5649, 61.5693) knots 0 0 0 1 2 2 2
  spline S930 degree 2 poles (-271.5649, 61.5693) (-271.5649, 61.8211) (-271.2084, 62.1832) (-270.9509, 62.1832) knots 0 0 0 1 2 2 2
  spline S931 degree 2 poles (-270.9509, 62.1832) (-270.6878, 62.1832) (-270.3285, 61.8154) (-270.3285, 61.5693) knots 0 0 0 1 2 2 2
  line L924 (-260.5391, 60.5309) -> (-260.6721, 61.0911)
  line L925 (-260.6721, 61.0911) -> (-261.5831, 61.0911)
  line L926 (-261.5831, 61.0911) -> (-261.7274, 60.5309)
  line L927 (-261.7274, 60.5309) -> (-262.7205, 60.5309)
  line L928 (-262.7205, 60.5309) -> (-261.6708, 63.5809)
  line L929 (-261.6708, 63.5809) -> (-260.5306, 63.5809)
  line L930 (-260.5306, 63.5809) -> (-259.5403, 60.5309)
  line L931 (-259.5403, 60.5309) -> (-260.5391, 60.5309)
  line L932 (-261.1163, 62.916) -> (-261.1361, 62.916)
  spline S932 degree 2 poles (-261.1361, 62.916) (-261.1417, 62.8651) (-261.1926, 62.6303) (-261.4247, 61.7447) knots 0 0 0 1 2 2 2
  line L933 (-261.4247, 61.7447) -> (-260.8418, 61.7447)
  line L934 (-260.8418, 61.7447) -> (-261.054, 62.5737)
  spline S933 degree 2 poles (-261.054, 62.5737) (-261.0993, 62.7576) (-261.1163, 62.916) knots 0 0 0 1 1 1
  line L935 (-259.2659, 60.5309) -> (-259.2659, 63.7563)
  line L936 (-259.2659, 63.7563) -> (-258.3605, 63.7563)
  line L937 (-258.3605, 63.7563) -> (-258.3605, 60.5309)
  line L938 (-258.3605, 60.5309) -> (-259.2659, 60.5309)
  spline S934 degree 2 poles (-256.247, 63.0971) (-256.3885, 63.1452) (-256.5073, 63.1452) knots 0 0 0 1 1 1
  spline S935 degree 2 poles (-256.5073, 63.1452) (-256.6601, 63.1452) (-256.8044, 62.9896) (-256.8044, 62.8594) knots 0 0 0 1 2 2 2
  line L939 (-256.8044, 62.8594) -> (-256.8044, 62.7095)
  line L940 (-256.8044, 62.7095) -> (-256.3008, 62.7095)
  line L941 (-256.3008, 62.7095) -> (-256.3008, 62.0814)
  line L942 (-256.3008, 62.0814) -> (-256.8044, 62.0814)
  line L943 (-256.8044, 62.0814) -> (-256.8044, 60.5309)
  line L944 (-256.8044, 60.5309) -> (-257.7098, 60.5309)
  line L945 (-257.7098, 60.5309) -> (-257.7098, 62.0814)
  line L946 (-257.7098, 62.0814) -> (-258.0747, 62.0814)
  line L947 (-258.0747, 62.0814) -> (-258.0747, 62.7095)
  line L948 (-258.0747, 62.7095) -> (-257.7098, 62.7095)
  line L949 (-257.7098, 62.7095) -> (-257.7098, 62.9104)
  spline S936 degree 2 poles (-257.7098, 62.9104) (-257.7098, 63.1763) (-257.4636, 63.5809) (-256.9939, 63.8073) (-256.6573, 63.8073) knots 0 0 0 1 2 3 3 3
  spline S937 degree 2 poles (-256.6573, 63.8073) (-256.4139, 63.8073) (-256.247, 63.7592) knots 0 0 0 1 1 1
  line L950 (-256.247, 63.7592) -> (-256.247, 63.0971)
  line L951 (-254.838, 60.5309) -> (-254.838, 60.8619)
  line L952 (-254.838, 60.8619) -> (-254.8465, 60.8619)
  spline S938 degree 2 poles (-254.8465, 60.8619) (-255.0644, 60.4772) (-255.5114, 60.4772) knots 0 0 0 1 1 1
  spline S939 degree 2 poles (-255.5114, 60.4772) (-255.8198, 60.4772) (-256.1678, 60.8421) (-256.1678, 61.1505) knots 0 0 0 1 2 2 2
  spline S940 degree 2 poles (-256.1678, 61.1505) (-256.1678, 61.7928) (-255.3784, 61.8946) knots 0 0 0 1 1 1
  line L953 (-255.3784, 61.8946) -> (-254.838, 61.9654)
  spline S941 degree 2 poles (-254.838, 61.9654) (-254.838, 62.0729) (-255.0304, 62.2087) (-255.1917, 62.2087) knots 0 0 0 1 2 2 2
  spline S942 degree 2 poles (-255.1917, 62.2087) (-255.5567, 62.2087) (-255.9641, 61.9993) knots 0 0 0 1 1 1
  line L954 (-255.9641, 61.9993) -> (-255.9641, 62.5878)
  spline S943 degree 2 poles (-255.9641, 62.5878) (-255.7887, 62.6642) (-255.2539, 62.7632) (-255.0644, 62.7632) knots 0 0 0 1 2 2 2
  spline S944 degree 2 poles (-255.0644, 62.7632) (-254.5098, 62.7632) (-254.009, 62.2879) (-254.009, 61.7334) knots 0 0 0 1 2 2 2
  line L955 (-254.009, 61.7334) -> (-254.009, 60.5309)
  line L956 (-254.009, 60.5309) -> (-254.838, 60.5309)
  spline S945 degree 2 poles (-255.3756, 61.2722) (-255.3756, 61.1845) (-255.2624, 61.0685) (-255.1577, 61.0685) knots 0 0 0 1 2 2 2
  spline S946 degree 2 poles (-255.1577, 61.0685) (-255.0163, 61.0685) (-254.838, 61.2807) (-254.838, 61.4476) knots 0 0 0 1 2 2 2
  line L957 (-254.838, 61.4476) -> (-254.838, 61.5297)
  line L958 (-254.838, 61.5297) -> (-255.1464, 61.4872)
  spline S947 degree 2 poles (-255.1464, 61.4872) (-255.3756, 61.4476) (-255.3756, 61.2722) knots 0 0 0 1 1 1
  line L959 (-252.1898, 60.5309) -> (-252.1898, 61.7192)
  spline S948 degree 2 poles (-252.1898, 61.7192) (-252.1898, 61.9229) (-252.3114, 62.0984) (-252.4472, 62.0984) knots 0 0 0 1 2 2 2
  spline S949 degree 2 poles (-252.4472, 62.0984) (-252.5632, 62.0984) (-252.6962, 61.9145) (-252.6962, 61.773) knots 0 0 0 1 2 2 2
  line L960 (-252.6962, 61.773) -> (-252.6962, 60.5309)
  line L961 (-252.6962, 60.5309) -> (-253.6016, 60.5309)
  line L962 (-253.6016, 60.5309) -> (-253.6016, 62.7095)
  line L963 (-253.6016, 62.7095) -> (-252.6962, 62.7095)
  line L964 (-252.6962, 62.7095) -> (-252.6962, 62.37)
  line L965 (-252.6962, 62.37) -> (-252.6877, 62.37)
  spline S950 degree 2 poles (-252.6877, 62.37) (-252.5802, 62.5567) (-252.2124, 62.7632) (-251.9974, 62.7632) knots 0 0 0 1 2 2 2
  spline S951 degree 2 poles (-251.9974, 62.7632) (-251.2844, 62.7632) (-251.2844, 61.8607) knots 0 0 0 1 1 1
  line L966 (-251.2844, 61.8607) -> (-251.2844, 60.5309)
  line L967 (-251.2844, 60.5309) -> (-252.1898, 60.5309)
  spline S952 degree 2 poles (-248.4522, 61.6598) (-248.4522, 61.1081) (-249.1171, 60.4772) (-249.7141, 60.4772) knots 0 0 0 1 2 2 2
  spline S953 degree 2 poles (-249.7141, 60.4772) (-250.3083, 60.4772) (-250.9703, 61.0911) (-250.9703, 61.6344) knots 0 0 0 1 2 2 2
  spline S954 degree 2 poles (-250.9703, 61.6344) (-250.9703, 61.9795) (-250.6591, 62.4916) (-250.0848, 62.7632) (-249.7113, 62.7632) knots 0 0 0 1 2 3 3 3
  spline S955 degree 2 poles (-249.7113, 62.7632) (-249.3237, 62.7632) (-248.755, 62.4775) (-248.4522, 61.971) (-248.4522, 61.6598) knots 0 0 0 1 2 3 3 3
  spline S956 degree 2 poles (-249.3718, 61.6542) (-249.3718, 62.0984) (-249.7113, 62.0984) knots 0 0 0 1 1 1
  spline S957 degree 2 poles (-249.7113, 62.0984) (-250.0508, 62.0984) (-250.0508, 61.6344) knots 0 0 0 1 1 1
  spline S958 degree 2 poles (-250.0508, 61.6344) (-250.0508, 61.142) (-249.7056, 61.142) knots 0 0 0 1 1 1
  spline S959 degree 2 poles (-249.7056, 61.142) (-249.3718, 61.142) (-249.3718, 61.6542) knots 0 0 0 1 1 1
  line L968 (-246.8197, 60.5309) -> (-246.8197, 63.5809)
  line L969 (-246.8197, 63.5809) -> (-244.9213, 63.5809)
  line L970 (-244.9213, 63.5809) -> (-244.9213, 62.8623)
  line L971 (-244.9213, 62.8623) -> (-245.9002, 62.8623)
  line L972 (-245.9002, 62.8623) -> (-245.9002, 62.4181)
  line L973 (-245.9002, 62.4181) -> (-244.9807, 62.4181)
  line L974 (-244.9807, 62.4181) -> (-244.9807, 61.6994)
  line L975 (-244.9807, 61.6994) -> (-245.9002, 61.6994)
  line L976 (-245.9002, 61.6994) -> (-245.9002, 61.2496)
  line L977 (-245.9002, 61.2496) -> (-244.8505, 61.2496)
  line L978 (-244.8505, 61.2496) -> (-244.8505, 60.5309)
  line L979 (-244.8505, 60.5309) -> (-246.8197, 60.5309)
  line L980 (-241.6732, 60.5309) -> (-241.6732, 61.7871)
  spline S960 degree 2 poles (-241.6732, 61.7871) (-241.6732, 61.9427) (-241.7864, 62.0984) (-241.9137, 62.0984) knots 0 0 0 1 2 2 2
  spline S961 degree 2 poles (-241.9137, 62.0984) (-242.0382, 62.0984) (-242.1797, 61.9088) (-242.1797, 61.7419) knots 0 0 0 1 2 2 2
  line L981 (-242.1797, 61.7419) -> (-242.1797, 60.5309)
  line L982 (-242.1797, 60.5309) -> (-243.085, 60.5309)
  line L983 (-243.085, 60.5309) -> (-243.085, 61.7645)
  spline S962 degree 2 poles (-243.085, 61.7645) (-243.085, 62.0984) (-243.3114, 62.0984) knots 0 0 0 1 1 1
  spline S963 degree 2 poles (-243.3114, 62.0984) (-243.45, 62.0984) (-243.5915, 61.906) (-243.5915, 61.7249) knots 0 0 0 1 2 2 2
  line L984 (-243.5915, 61.7249) -> (-243.5915, 60.5309)
  line L985 (-243.5915, 60.5309) -> (-244.4969, 60.5309)
  line L986 (-244.4969, 60.5309) -> (-244.4969, 62.7095)